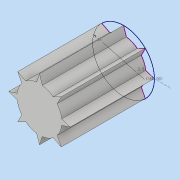
# Autodesk Inventor part: 滚轮设计
Saved by Autodesk Inventor 2019 (Build 230136000, 136)
## iProperties
Created: 2020-11-01
Part Number: 滚轮设计
Material: Generic
Document SubType Name: Modeling
Designer: Wang Hua
Density: 1 g/cm^3
Appearance: Default
Author: Wang Hua
Autodesk Inventor part; units mm, degrees
ref_plane "YZ Plane" through (0, 0, 0) normal (1, 0, 0) x (0, 1, 0)
ref_plane "XZ Plane" through (0, 0, 0) normal (0, 1, 0) x (-1, 0, 0)
ref_plane "XY Plane" through (0, 0, 0) normal (0, 0, 1) x (1, 0, 0)
sketch "草图1" plane through (0, 0, 0) normal (0, 0, 1) x (1, 0, 0)
  circle A0 centre (0, 0) radius 27.5
  line L0 (27.5, 0) -> (19.8431, 2.5)
  line L1 (0, 0) -> (42.7409, 0) construction
  line L2 (27.5, 0) -> (19.8431, -2.5)
  line L3 (19.4454, 19.4454) -> (12.2634, 15.799)
  line L4 (19.4454, 19.4454) -> (15.799, 12.2634)
  line L5 (0, 27.5) -> (-2.5, 19.8431)
  line L6 (0, 27.5) -> (2.5, 19.8431)
  line L7 (-19.4454, 19.4454) -> (-15.799, 12.2634)
  line L8 (-19.4454, 19.4454) -> (-12.2634, 15.799)
  line L9 (-27.5, 0) -> (-19.8431, -2.5)
  line L10 (-27.5, 0) -> (-19.8431, 2.5)
  line L11 (-19.4454, -19.4454) -> (-12.2634, -15.799)
  line L12 (-19.4454, -19.4454) -> (-15.799, -12.2634)
  line L13 (0, -27.5) -> (2.5, -19.8431)
  line L14 (0, -27.5) -> (-2.5, -19.8431)
  line L15 (19.4454, -19.4454) -> (15.799, -12.2634)
  line L16 (19.4454, -19.4454) -> (12.2634, -15.799)
  arc A1 (19.8431, 2.5) -> (15.799, 12.2634) centre (0, 0) ccw
  arc A2 (15.799, -12.2634) -> (19.8431, -2.5) centre (0, 0) ccw
  arc A3 (2.5, -19.8431) -> (12.2634, -15.799) centre (0, 0) ccw
  arc A4 (-12.2634, -15.799) -> (-2.5, -19.8431) centre (0, 0) ccw
  arc A5 (-19.8431, -2.5) -> (-15.799, -12.2634) centre (0, 0) ccw
  arc A6 (-15.799, 12.2634) -> (-19.8431, 2.5) centre (0, 0) ccw
  arc A7 (12.2634, 15.799) -> (2.5, 19.8431) centre (0, 0) ccw
  arc A8 (-2.5, 19.8431) -> (-12.2634, 15.799) centre (0, 0) ccw
  dimension "d1" = 55
  dimension "d2" = 2.5
  dimension "d5" = 360
  constraints: 34 end point, 16 point on circle, 8 centre point, 2 coincident, 1 horizontal, 1 horizontal alignment, 1 point on line, 1 symmetric about line, 43 other
  measures "d2" vertical distance of L0.start L0.end
extrude "拉伸1" add sketch "草图1" along normal blind 75 contours L2 A2 L15 L16 A3 L13 L14 A4 L11 L12 A5 L9 L10 A6 L7 L8 A8 L5 L6 A7 L3 L4 A1 L0
